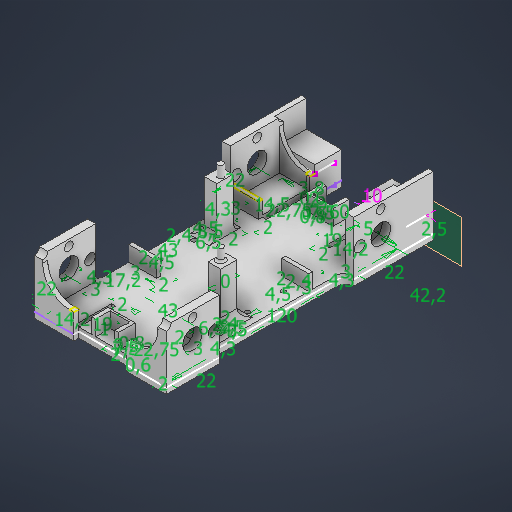
# Autodesk Inventor part: MainBody_thin
Saved by Autodesk Inventor 2026.1 (Build 301233000, 233)
## iProperties
Created: 2026-05-04
Part Number: MainBody_thin
Material: Generic
Document SubType Name: Modeling
Designer: 25adoh
Density: 1 g/cm^3
Appearance: Default
Author: 25adoh
Autodesk Inventor part; units mm, degrees
ref_plane "YZ Plane" through (0, 0, 0) normal (1, 0, 0) x (0, 1, 0)
ref_plane "XZ Plane" through (0, 0, 0) normal (0, 1, 0) x (-1, 0, 0)
ref_plane "XY Plane" through (0, 0, 0) normal (0, 0, 1) x (1, 0, 0)
sketch "Sketch1" plane through (0, 0, 0) normal (0, 1, 0) x (-1, 0, 0)
  line L0 (0, 0) -> (-60, 0)
  line L1 (-60, 0) -> (-60, -120)
  line L2 (-60, -120) -> (0, -120)
  line L3 (0, -120) -> (0, 0)
  line L4 (0, 0) -> (4.3, 0)
  line L5 (4.3, 0) -> (4.3, -22)
  line L6 (4.3, -22) -> (0, -22)
  line L7 (0, -22) -> (0, 0)
  line L8 (-60, 0) -> (-64.3, 0)
  line L9 (-64.3, 0) -> (-64.3, -22)
  line L10 (-64.3, -22) -> (-60, -22)
  line L11 (-60, -22) -> (-60, 0)
  line L12 (0, -120) -> (4.3, -120)
  line L13 (4.3, -120) -> (4.3, -98)
  line L14 (4.3, -98) -> (0, -98)
  line L15 (0, -98) -> (0, -120)
  line L16 (-60, -120) -> (-64.3, -120)
  line L17 (-64.3, -120) -> (-64.3, -98)
  line L18 (-64.3, -98) -> (-60, -98)
  line L19 (-60, -98) -> (-60, -120)
  line L20 (-45.8, -101.0095) -> (-43.8, -101.0095)
  line L21 (-43.8, -101.0095) -> (-43.8, -120)
  line L22 (-14.2, 0) -> (-14.2, -19)
  line L23 (-14.2, -19) -> (-16.2, -19)
  line L24 (-16.2, -19) -> (-16.2, 0)
  line L25 (-16.2, 0) -> (-14.2, 0)
  line L26 (-16.5, -120) -> (-14.5, -120)
  line L27 (-45.2, -120) -> (-43.8, -120)
  line L28 (-46, -77.8) -> (-60, -77.8)
  line L29 (-46, -77.8) -> (-46, -75.8)
  line L30 (-46, -75.8) -> (-60, -75.8)
  line L31 (0, 0) -> (-14.2, 0)
  line L32 (-14.5, -42.2) -> (0, -42.2)
  line L33 (-43.5, 0) -> (-43.5, -22.75)
  line L34 (-45.5, 0) -> (-45.5, -22.75)
  line L35 (-45.5, -22.75) -> (-43.5, -22.75)
  line L36 (-43.5, -22.75) -> (-43.5, -24.75)
  line L37 (-43.5, 0) -> (-45.5, 0)
  line L38 (-43.5, -24.75) -> (-60, -24.75)
  line L39 (-45.5, -22.75) -> (-60, -22.75)
  line L40 (-14.5, -120) -> (-14.5, -97.25)
  line L41 (-14.5, -97.25) -> (0, -97.25)
  line L42 (-16.5, -120) -> (-16.5, -97.25)
  line L43 (-16.5, -97.25) -> (-14.5, -97.25)
  line L44 (-16.5, -97.25) -> (-16.5, -95.25)
  line L45 (-16.5, -95.25) -> (0, -95.25)
  line L46 (-45.5, 0) -> (-45.5, 0.6)
  line L47 (-60, 0) -> (-60, 0.6)
  line L48 (-60, 0.6) -> (-45.5, 0.6)
  line L49 (-60, 0.6) -> (-60, 2.6)
  line L50 (-60, 2.6) -> (-43.5, 2.6)
  line L51 (-43.5, 2.6) -> (-43.5, 0)
  line L52 (-16.5, -120) -> (-16.5, -120.6)
  line L53 (-16.5, -120.6) -> (0, -120.6)
  line L54 (-16.5, -120.6) -> (-16.5, -122.6)
  line L55 (-16.5, -122.6) -> (0, -122.6)
  line L56 (0, -122.6) -> (0, -120.6)
  line L57 (0, -120.6) -> (0, -120)
  line L58 (-14.5, -120) -> (-14.5, -120.6)
  line L59 (-16.2, 0) -> (0, 0)
  line L60 (0, 0) -> (0, 2.6)
  line L61 (0, 2.6) -> (-16.2, 2.6)
  line L62 (-16.2, 2.6) -> (-16.2, 0)
  line L63 (-43.8, -120) -> (-59.8, -120)
  line L64 (-59.8, -120) -> (-59.8, -122.6)
  line L65 (-59.8, -122.6) -> (-43.8, -122.6)
  line L66 (-43.8, -122.6) -> (-43.8, -120)
  line L67 (-45.8, -101.0095) -> (-45.8, -120)
  line L68 (-14.5, -42.2) -> (-14.5, -44.2)
  line L69 (-14.5, -44.2) -> (0, -44.2)
  line L70 (-35, -120) -> (-35, 0)
  line L71 (-64.3, -22) -> (-60, -22)
  line L72 (-60, -22) -> (-60, -25)
  line L73 (-60, -25) -> (-64.3, -25)
  line L74 (-64.3, -25) -> (-64.3, -22)
  line L75 (-64.3, -98) -> (-60, -98)
  line L76 (-60, -98) -> (-60, -95)
  line L77 (-60, -95) -> (-64.3, -95)
  line L78 (-64.3, -95) -> (-64.3, -98)
  line L79 (4.3, -22) -> (0, -22)
  line L80 (0, -22) -> (0, -25)
  line L81 (0, -25) -> (4.3, -25)
  line L82 (4.3, -25) -> (4.3, -22)
  line L83 (4.3, -98) -> (0, -98)
  line L84 (0, -98) -> (0, -95)
  line L85 (0, -95) -> (4.3, -95)
  line L86 (4.3, -95) -> (4.3, -98)
  line L87 (-64.3, 0) -> (-60, 0)
  line L88 (-60, 0) -> (-60, 2.6)
  line L89 (-60, 2.6) -> (-64.3, 2.6)
  line L90 (-64.3, 2.6) -> (-64.3, 0)
  line L91 (0, 2.6) -> (4.3, 2.6)
  line L92 (4.3, 2.6) -> (4.3, 0)
  line L93 (4.3, 0) -> (0, 0)
  line L94 (0, 0) -> (0, 2.6)
  line L95 (0, -122.6) -> (4.3, -122.6)
  line L96 (4.3, -122.6) -> (4.3, -120)
  line L97 (4.3, -120) -> (0, -120)
  line L98 (0, -120) -> (0, -122.6)
  line L99 (-64.3, -120) -> (-59.8, -120)
  line L100 (-59.8, -120) -> (-59.8, -122.6)
  line L101 (-59.8, -122.6) -> (-64.3, -122.6)
  line L102 (-64.3, -122.6) -> (-64.3, -120)
  line L103 (-25, 0) -> (-35, 0)
  line L104 (-35, 0) -> (-35, -7.5)
  line L105 (-35, -7.5) -> (-25, -7.5)
  line L106 (-25, -7.5) -> (-25, 0)
  line L107 (-35, -7.5) -> (-35, -6.7)
  line L108 (-35, -5.7) -> (-35, -6.7)
  line L109 (-25, 0) -> (-23, 0)
  line L110 (-35, -7.5) -> (-37, -7.5)
  line L111 (-37, -7.5) -> (-37, 0)
  line L112 (-37, 0) -> (-35, 0)
  line L113 (-35, 0) -> (-35, -7.5)
  line L114 (-35, -6.7) -> (-35.3, -6.7)
  line L115 (-35, -6.5) -> (-35, -6.7)
  line L116 (-37, -7.5) -> (-23, -7.5)
  line L117 (-23, -8.5) -> (-37, -8.5)
  line L118 (-37, -8.5) -> (-37, -7.5)
  line L119 (-35, -6.7) -> (-35.5, -6.7)
  line L120 (-35.5, -6.7) -> (-35.5, -5.7)
  line L121 (-35.5, -5.7) -> (-35, -5.7)
  line L122 (-35, -5.7) -> (-35, -6.7)
  line L123 (-14.2, 0) -> (0, 0)
  line L124 (0, -25) -> (0, -42.2)
  line L125 (-23, -8.5) -> (-23, 0)
  line L126 (-25, -120) -> (-25, 0)
  circle A0 centre (-7, -69) radius 1.2
  circle A1 centre (-7, -51) radius 1.2
  circle A2 centre (-53.3, -50.7) radius 1.2
  circle A3 centre (-53.3, -69.3) radius 1.2
  line L127 (-51.5, -81.5) -> (-8.5, -81.5)
  line L128 (-8.5, -81.5) -> (-8.5, -38.5)
  line L129 (-8.5, -38.5) -> (-51.5, -38.5)
  line L130 (-51.5, -38.5) -> (-51.5, -81.5)
  line L131 (-51.5, -81.5) -> (-8.5, -38.5) construction
  line L132 (-8.5, -81.5) -> (-51.5, -38.5) construction
  circle A4 centre (-11.25, -41.25) radius 1.5
  circle A5 centre (-11.25, -41.25) radius 2.25
  line L133 (-9, -43.5) -> (-13.5, -43.5)
  line L134 (-13.5, -43.5) -> (-13.5, -39)
  line L135 (-13.5, -39) -> (-9, -39)
  line L136 (-9, -39) -> (-9, -43.5)
  circle A6 centre (-48.75, -41.25) radius 1.5
  circle A7 centre (-48.75, -41.25) radius 2.25
  line L137 (-51, -43.5) -> (-46.5, -43.5)
  line L138 (-46.5, -43.5) -> (-46.5, -39)
  line L139 (-46.5, -39) -> (-51, -39)
  line L140 (-51, -39) -> (-51, -43.5)
  circle A8 centre (-48.75, -78.75) radius 1.5
  circle A9 centre (-48.75, -78.75) radius 2.25
  line L141 (-46.5, -76.5) -> (-51, -76.5)
  line L142 (-51, -76.5) -> (-51, -81)
  line L143 (-51, -81) -> (-46.5, -81)
  line L144 (-46.5, -81) -> (-46.5, -76.5)
  circle A10 centre (-11.25, -78.75) radius 1.5
  circle A11 centre (-11.25, -78.75) radius 2.25
  line L145 (-13.5, -76.5) -> (-9, -76.5)
  line L146 (-9, -76.5) -> (-9, -81)
  line L147 (-9, -81) -> (-13.5, -81)
  line L148 (-13.5, -81) -> (-13.5, -76.5)
  line L149 (-14.5, -97.25) -> (-14.5, -95.25)
  line L150 (-45.5, -22.75) -> (-45.5, -24.75)
  line L151 (-46.5, -70.3) -> (-51, -70.3)
  line L152 (-51, -70.3) -> (-51, -65.8)
  line L153 (-51, -65.8) -> (-46.5, -65.8)
  line L154 (-46.5, -65.8) -> (-46.5, -70.3)
  line L155 (-13.5, -49.7) -> (-9, -49.7)
  line L156 (-9, -49.7) -> (-9, -54.2)
  line L157 (-9, -54.2) -> (-13.5, -54.2)
  line L158 (-13.5, -54.2) -> (-13.5, -49.7)
  line L159 (-25, -120) -> (-25, -112.5)
  line L160 (-25, -112.5) -> (-35, -112.5)
  line L161 (-35, -112.5) -> (-35, -120)
  line L162 (-25, -112.5) -> (-25, -113.3)
  line L163 (-25, -114.3) -> (-25, -113.3)
  line L164 (-35, -120) -> (-37, -120)
  line L165 (-25, -112.5) -> (-23, -112.5)
  line L166 (-23, -112.5) -> (-23, -120)
  line L167 (-23, -120) -> (-25, -120)
  line L168 (-25, -120) -> (-25, -112.5)
  line L169 (-25, -113.3) -> (-24.7, -113.3)
  line L170 (-25, -113.5) -> (-25, -113.3)
  line L171 (-23, -112.5) -> (-37, -112.5)
  line L172 (-37, -111.5) -> (-23, -111.5)
  line L173 (-23, -111.5) -> (-23, -112.5)
  line L174 (-25, -113.3) -> (-24.5, -113.3)
  line L175 (-24.5, -113.3) -> (-24.5, -114.3)
  line L176 (-24.5, -114.3) -> (-25, -114.3)
  line L177 (-25, -114.3) -> (-25, -113.3)
  line L178 (-37, -111.5) -> (-37, -120)
  line L179 (-30, -60) -> (-30, -60)
  line L180 (-30, -60) -> (-30, -60)
  line L181 (-30, -60) -> (-30, -60)
  line L182 (-53.3, -120) -> (-53.1894, -77.8)
  line L183 (-64.3, -122.6) -> (-42.6503, -122.6)
  line L184 (-64.3, -122.6) -> (-59.3, -122.6)
  line L185 (-47.6503, -122.6) -> (-42.6503, -122.6)
  line L186 (4.3, -122.6) -> (-16.5, -122.6)
  line L187 (4.3, -132.6) -> (4.3, -122.6)
  line L188 (-16.5, -122.6) -> (-11.5, -122.6)
  line L189 (4.3, -122.6) -> (-0.7, -122.6)
  line L190 (4.3, -132.6) -> (4.3, -122.6)
  line L191 (-46.5, -43.5) -> (-46.5, -45.5)
  line L192 (-46.5, -45.5) -> (-53, -45.5)
  line L193 (-53, -45.5) -> (-53, -37)
  line L194 (-53, -37) -> (-46.5, -37)
  line L195 (-46.5, -37) -> (-46.5, -45.5)
  line L196 (-13.5, -81) -> (-13.5, -83)
  line L197 (-13.5, -83) -> (-7, -83)
  line L198 (-7, -83) -> (-7, -74.5)
  line L199 (-7, -74.5) -> (-13.5, -74.5)
  line L200 (-13.5, -74.5) -> (-13.5, -83)
  line L201 (-64.3, -120) -> (4.3, -120)
  line L202 (4.3, -120) -> (4.3, -136.4)
  line L203 (-0.7, -122.6) -> (-11.5, -122.6)
  line L204 (-11.5, -122.6) -> (-11.5, -126.4)
  line L205 (-11.5, -126.4) -> (-0.7, -126.4)
  line L206 (-0.7, -126.4) -> (-0.7, -122.6)
  line L207 (-16.5, -136.4) -> (-11.5, -136.4)
  line L208 (-11.5, -136.4) -> (-11.5, -122.6)
  line L209 (-11.5, -122.6) -> (-16.5, -122.6)
  line L210 (-16.5, -122.6) -> (-16.5, -136.4)
  line L211 (4.3, -136.4) -> (-0.7, -136.4)
  line L212 (-0.7, -136.4) -> (-0.7, -122.6)
  line L213 (-0.7, -122.6) -> (4.3, -122.6)
  line L214 (4.3, -122.6) -> (4.3, -136.4)
  line L215 (-0.7, -136.4) -> (-11.5, -136.4)
  line L216 (-64.3, -122.6) -> (-59.8, -122.6)
  line L217 (-59.8, -122.6) -> (-59.8, -136.4)
  line L218 (-59.8, -136.4) -> (-64.3, -136.4)
  line L219 (-64.3, -136.4) -> (-64.3, -122.6)
  line L220 (-42.6503, -122.6) -> (-47.6503, -122.6)
  line L221 (-47.6503, -122.6) -> (-47.6503, -136.4)
  line L222 (-47.6503, -136.4) -> (-42.6503, -136.4)
  line L223 (-42.6503, -136.4) -> (-42.6503, -122.6)
  line L224 (-47.6503, -136.4) -> (-59.8, -136.4)
  line L225 (-47.6503, -126.4) -> (-59.8, -126.4)
  line L226 (-42.6503, -122.6) -> (-42.6503, -120)
  line L227 (-64.3, -120) -> (-61.8, -120)
  line L228 (-61.8, -120) -> (-61.8, -136.4)
  line L229 (-61.8, -136.4) -> (-64.3, -136.4)
  line L230 (-64.3, -136.4) -> (-64.3, -120)
  line L231 (4.3, -122.6) -> (1.8, -122.6)
  line L232 (1.8, -122.6) -> (1.8, -136.4)
  line L233 (1.8, -136.4) -> (4.3, -136.4)
  line L234 (4.3, -136.4) -> (4.3, -122.6)
  line L235 (1.8, -122.6) -> (4.3, -122.6)
  line L236 (4.3, -122.6) -> (4.3, -120)
  line L237 (4.3, -120) -> (1.8, -120)
  line L238 (1.8, -120) -> (1.8, -122.6)
  point P0 (-60, -98)
  point P1 (0, -98)
  point P2 (0, -29.2)
  point P3 (-35, -130)
  point P4 (-45.8, -120)
  point P5 (-60, -120)
  point P6 (-30, -70)
  point P7 (-30, -60)
  point P8 (-30, -60)
  point P9 (-12.75, -42.75)
  point P10 (-35, -8.5)
  point P11 (-25, -120)
  point P12 (-37, -120)
  point P13 (-35, -112.5)
  point P14 (-25, -112.5)
  point P15 (-25, -113.3)
  point P16 (-25, -114.3)
  point P17 (-23, -120)
  point P18 (-25, -120)
  point P19 (-25, -111.5)
  point P20 (-25, -112.5)
  point P21 (-25, -120)
  point P22 (-35, -111.5)
  point P23 (-16.5, -132.6)
  point P24 (-51, -41.25)
  point P25 (-43.8, -122.6)
  point P26 (-0.7, -126.4)
  point P27 (-0.7, -122.6)
  dimension "d0" = 60
  dimension "d1" = 120
  dimension "d2" = 4.3
  dimension "d3" = 22
  dimension "d4" = 4.3
  dimension "d5" = 22
  dimension "d6" = 4.3
  dimension "d7" = 22
  dimension "d8" = 4.3
  dimension "d9" = 22
  dimension "d66" = 19
  dimension "d67" = 2
  dimension "d74" = 19
  dimension "d75" = 2
  dimension "d100" = 2
  dimension "d107" = 22.75
  dimension "d108" = 2
  dimension "d109" = 22.75
  dimension "d110" = 2
  dimension "d111" = 0.6
  dimension "d112" = 2
  dimension "d113" = 0.6
  dimension "d114" = 2
  dimension "d148" = 2
  dimension "d165" = 3
  dimension "d166" = 3
  dimension "d167" = 3
  dimension "d168" = 3
  dimension "d175" = 7.5
  dimension "d176" = 0.8
  dimension "d180" = 2
  dimension "d182" = 1
  dimension "d183" = 0.5
  dimension "d186" = 14.2
  dimension "d190" = 17.2
  dimension "d196" = 2.4
  dimension "d197" = 2.4
  dimension "d198" = 2.4
  dimension "d199" = 43
  dimension "d200" = 43
  dimension "d201" = 3
  dimension "d202" = 3
  dimension "d203" = 4.5
  dimension "d204" = 3
  dimension "d205" = 4.5
  dimension "d206" = 4.5
  dimension "d207" = 4.5
  dimension "d209" = 2.4
  dimension "d215" = 7.5
  dimension "d216" = 0.8
  dimension "d217" = 2
  dimension "d218" = 1
  dimension "d219" = 0.5
  dimension "d224" = 0
  dimension "d225" = 42.2
  dimension "d228" = 5
  dimension "d238" = 2
  dimension "d239" = 6.5
  dimension "d240" = 8.5
  dimension "d241" = 2
  dimension "d242" = 6.5
  dimension "d243" = 8.5
  dimension "d247" = 14.2
  dimension "d248" = 14.5
  constraints: 474 end point, 79 parallel, 57 perpendicular, 53 horizontal, 27 point on line, 20 vertical, 12 centre point, 4 coincident, 4 midpoint, 3 collinear, 20 other
  measures "d0" distance of L2.end L1.end
  measures "d1" distance of L1.end L1.start
  measures "d2" distance of L5.end L6.end
  measures "d3" distance of L4.end L5.end
  measures "d4" distance of L10.end L9.end
  measures "d5" distance of L9.end L8.end
  measures "d6" distance of L14.end L13.end
  measures "d7" distance of L13.end L12.end
  measures "d8" distance of L17.end L18.end
  measures "d9" distance of L16.end L17.end
  measures "d66" distance of L27.start L20.start
  measures "d67" distance of L20.start L20.end
  measures "d74" distance of L22.start L22.end
  measures "d75" distance of L22.end L23.end
  measures "d100" distance of L28.start L29.end
  measures "d107" distance of L33.start L33.end
  measures "d108" distance of L33.end L36.end
  measures "d109" distance of L26.end L40.end
  measures "d110" distance of L42.end L44.end
  measures "d111" distance of L34.start L46.end
  measures "d112" distance of L47.end L49.end
  measures "d113" distance of L26.start L52.end
  measures "d114" distance of L52.end L54.end
  measures "d148" distance of L32.start L68.end
  measures "d165" distance of L71.end L72.end
  measures "d166" distance of L76.end L75.end
  measures "d167" distance of L80.end L79.end
  measures "d168" distance of L83.end L84.end
  measures "d175" distance of L104.end L103.end
  measures "d176" distance of L104.end L107.end
  measures "d180" distance of L111.end L112.end
  measures "d182" distance of L116.end L117.start
  measures "d183" distance of L120.end L121.end
  measures "d186" distance of L4.start L22.start
  measures "d190" distance of L80.end L32.end
  measures "d196" diameter of A0
  measures "d197" diameter of A2
  measures "d198" diameter of A3
  measures "d199" distance of L129.end L128.end
  measures "d200" distance of L128.end L127.end
  measures "d201" diameter of A4
  measures "d202" diameter of A6
  measures "d203" diameter of A7
  measures "d204" diameter of A8
  measures "d205" diameter of A11
  measures "d206" distance of L151.end L152.end
  measures "d207" distance of L155.end L156.end
  measures "d209" diameter of A1
  measures "d215" distance of L160.start L159.start
  measures "d216" distance of L160.start L177.end
  measures "d217" distance of L167.start L168.start
  measures "d218" distance of L171.end L178.start
  measures "d219" distance of L175.end L177.start
  measures "d224" distance of L180.end L181.end
  measures "d225" vertical distance of L182.start L182.end
  measures "d228" distance of L185.start L185.end
  measures "d238" distance of L137.end L191.end
  measures "d239" distance of L193.end L194.end
  measures "d240" distance of L192.end L193.end
  measures "d241" distance of L148.start L196.end
  measures "d242" distance of L199.end L198.end
  measures "d243" distance of L198.end L197.end
  measures "d247" distance between parallel lines of L67 L1
  measures "d248" distance between parallel lines of L40 L15
extrude "Extrusion1" add sketch "Sketch1" along normal blind 2 and the other way blind 3 contours L3 L32 L128 L129 L126 L117 L125 L0 L24 L23 L22 | L22 L23 L24 L0 | L125 L116 L106 L0 | L3 L69 L128 L32 | L106 L105 L70 L0 | L125 L117 L126 L116 | L3 L45 L44 L42 L2 L166 L173 L172 L126 L127 L196 L197 L198 L199 L128 L69 | L128 L69 L68 L32 L134 L133 L136 | L32 L136 L135 L134 L68 L69 L128 L199 L200 L148 L196 L127 L126 L129 | L70 L121 L120 L119 L114 L110 L111 L0 | L126 L117 L70 L105 | L136 L133 A5 L32 | L32 A5 L136 | L111 L118 L117 L70 L129 L195 L194 L193 L192 L130 L30 L1 L38 L36 L33 L0 | L70 L114 L119 L120 L121 | L70 L117 L118 L110 | L126 L129 L70 L117 | L3 L41 L149 L45 | L199 L198 L197 L196 L127 L128 | L128 L127 L196 L147 L146 L145 L200 L199 | A5 L32 A4 | L32 A4 A5 | A5 L135 L136 | L126 L127 L70 L129 | L33 L35 L34 L0 | L0 L46 L48 L49 L50 L51 | L3 L2 L40 L41 | L149 L43 L44 L45 | A4 L32 | L32 A4 | L133 L134 L32 A5 | A5 L134 L135 | L126 L172 L70 L127 | L70 L127 L130 L28 L142 L143 L144 L29 L30 L192 L191 L138 L195 L129 | L34 L39 L1 L0 | L0 L47 L48 L46 | L36 L38 L150 L35 | L40 L2 L42 L43 | L134 A5 L32 | L145 A11 L148 | L172 L173 L165 L126 | L126 L160 L70 L172 | L70 L172 L178 L2 L21 L20 L67 L182 L28 L130 L127 | L195 L139 L140 L137 L191 L192 L130 L129 | L129 L130 L192 L193 L194 L195 | L150 L38 L1 L39 | L57 L53 L58 L2 | L58 L53 L52 L2 | L187 L202 L211 L232 L95 | L148 A11 L147 | L145 L146 A11 | A11 | L165 L166 L2 L126 L176 L175 L174 L169 | L126 L2 L70 L160 | L70 L171 L178 L172 | L138 A7 L139 | L56 L55 L54 L53 | L232 L211 L212 L206 L55 L95 | A11 L146 L147 | L169 L174 L175 L176 L126 | L70 L2 L178 L171 | L130 L30 L29 L28 L144 L141 L142 | L28 L1 L30 L130 | A7 | L138 L137 A7 | A7 L140 L139 | L142 L141 A9 L28 | L28 A9 L142 | L182 L2 L1 L28 | L137 L140 A7 | L55 L204 L208 L207 L210 | A9 L28 A8 | L28 A8 A9 | A9 L143 L142 | A8 L28 | L28 A8 | L141 L144 L28 A9 | A9 L144 L143 | L67 L20 L21 L2 | L223 L222 L221 L65 L183 | L28 L144 A9 | L217 L218 L228 L101 | L228 L218 L219 L101 | A0 | A1 | A2 | A3 | A6 | A10 | L151 L152 L153 L154 | L155 L156 L157 L158
extrude "Extrusion2" add sketch "Sketch1" along normal blind 28 and the other way blind 3 contours L4 L5 L6 L3 | L6 L82 L81 L3 | L85 L86 L14 L3 | L13 L12 L3 L14 | L96 L95 L238 L12 | L1 L10 L9 L8 | L187 L202 L211 L232 L95 | L1 L73 L74 L10 | L1 L18 L78 L77 | L1 L16 L17 L18 | L228 L101 L102 L16 | L228 L218 L219 L101
sketch "Sketch2" plane through (64.3, -3, 0) normal (1, 0, 0) x (0, 0, -1)
  line L0 (0, 31) -> (25, 31) projected
  line L1 (22, 0) -> (22, 28) projected
  line L2 (0, 31) -> (0, 8)
  line L3 (0, 8) -> (22, 8)
  line L4 (0, 31) -> (22, 8)
  line L5 (22, 0) -> (22, 28) projected
  line L6 (0, 8) -> (22, 28)
  circle A0 centre (11, 18) radius 5.1
  line L7 (98, 28) -> (120, 28)
  line L8 (98, 0) -> (98, 28)
  line L9 (120, 0) -> (120, 28)
  line L10 (98, 28) -> (98, 5)
  line L11 (98, 5) -> (120, 5)
  line L12 (98, 28) -> (120, 5)
  line L13 (120, 0) -> (120, 28)
  line L14 (98, 5) -> (120, 28)
  circle A1 centre (109, 16.5) radius 5.1
  line L15 (120, 31) -> (120, 0) projected
  line L16 (0, 31) -> (0, 8)
  line L17 (12.5, 31) -> (11.25, 31) construction
  circle A2 centre (11, 27.75) radius 2.25
  circle A3 centre (109, 27.75) radius 2.25
  circle A4 centre (22, 16.5) radius 2.75
  circle A5 centre (98, 16.5) radius 2.75
  point P0 (118, 16.5)
  dimension "d14" = 23
  dimension "d15" = 10.2
  dimension "d16" = 23
  dimension "d17" = 10.2
  dimension "d60" = 4.5
  dimension "d61" = 4.5
  dimension "d115" = 5.5
  dimension "d214" = 5.5
  constraints: 28 end point, 6 centre point, 4 point on line, 3 midpoint, 3 perpendicular, 1 coincident, 1 horizontal, 2 other
  measures "d14" distance of L2.start L2.end
  measures "d15" diameter of A0
  measures "d16" distance of L7.start L10.end
  measures "d17" diameter of A1
  measures "d60" diameter of A2
  measures "d61" diameter of A3
  measures "d115" diameter of A4
  measures "d214" diameter of A5
extrude "Extrusion3" cut sketch "Sketch2" against normal up to surface (68.6 mm away) contours A4 L1 | L1 A4 | A0 L6 L4 | L4 L6 A0 | A0 L4 L6 | L4 A0 L6 | A3 L7 | L7 A3 | A5 L8 | L8 A5 | A1 L14 L12 | L12 L14 A1 | L14 A1 L12 | L12 A1 L14 | A2
ref_plane "Work Plane1" through (64.5, 0, -140) normal (0, 0, -1) x (-1, 0, 0)
sketch "Sketch5" plane through (64.5, 0, -140) normal (0, 0, -1) x (-1, 0, 0)
  line L0 (42, 5) -> (42, 20) projected
  line L1 (4.5, 2) -> (4.5, 28) projected
  line L2 (2.7, 28) -> (4.5, 28) projected
  line L3 (34.5, 20) -> (34.5, 5)
  line L4 (27, 5) -> (42, 5) projected
  line L5 (34.5, 5) -> (34.5, 13)
  line L6 (30.5, 13) -> (38.5, 13)
  line L7 (38.5, 13) -> (38.5, 5)
  line L8 (30.5, 13) -> (30.5, 5)
  line L9 (48, -3) -> (48, 2) projected
  line L10 (4.5, 2) -> (48, 2) projected
  line L11 (48, -3) -> (2.7, -3) projected
  line L12 (2.7, 28) -> (2.7, -3) projected
  point P0 (64.5, 0)
  point P1 (42, 5)
  dimension "d40" = 8
  dimension "d41" = 8
  constraints: 10 end point, 3 point on line, 2 midpoint, 2 perpendicular, 1 horizontal
  measures "d40" distance of L3.end L5.end
  measures "d41" distance of L6.start L6.end
extrude "Extrusion6" cut sketch "Sketch5" against normal blind 6 contours L6 L7 L4 L3 | L3 L4 L8 L6
extrude "Extrusion7" add sketch "Sketch1" along normal blind 10 and the other way blind 3 contours L60 L91 L92 L4 | L0 L62 L61 L60 | L3 L69 L128 L32 | L128 L69 L68 L32 L134 L133 L136 | L136 L133 A5 L32 | L3 L41 L149 L45 | A5 L32 A4 | L0 L46 L48 L49 L50 L51 | A4 L32 | L133 L134 L32 A5 | L96 L95 L238 L12 | L8 L90 L89 L49 L47 | L150 L38 L1 L39 | L12 L238 L95 L56 L57 | L58 L53 L52 L2 | L56 L55 L54 L53 | L130 L30 L29 L28 L144 L141 L142 | L28 L1 L30 L130 | L142 L141 A9 L28 | A9 L28 A8 | L2 L66 L65 L64 | A8 L28 | L141 L144 L28 A9 picked at (-12.908, -42.3449) picked at (-10.942, -42.2772) picked at (-50.408, -77.6551) picked at (-49.043, -77.5876)
extrude "Extrusion8" add sketch "Sketch1" along normal blind 28 contours L199 L198 L197 L196 L127 L128 | L128 L127 L196 L147 L146 L145 L200 L199 | L145 A11 L148 | L195 L139 L140 L137 L191 L192 L130 L129 | L129 L130 L192 L193 L194 L195 | L148 A11 L147 | L145 L146 A11 | A11 | L138 A7 L139 | A11 L146 L147 | A7 | L138 L137 A7 | A7 L140 L139 | L137 L140 A7 | A6 | A10
extrude "Extrusion9" add sketch "Sketch1" along normal blind 34 contours A6 | A10
fillet "Fillet3" radius 4.5 4 edges at (0, -0.5, -25) (0, -0.5, -95) (60, -0.5, -95) (60, -0.5, -25)
extrude "Extrusion12" add sketch "Sketch1" along normal blind 3 contours L3 L2 L40 L41 | L34 L39 L1 L0 | L0 L47 L48 L46 | L57 L53 L58 L2
extrude "Extrusion14" cut sketch "Sketch1" along normal blind 5 and the other way blind 5 contours A0 | A1 | A2 | A3
fillet "Fillet4" radius 1.5 4 edges at (54.5, -3, -50.7) (54.5, -3, -69.3) (8.2, -3, -51) (8.2, -3, -69)
fillet "Fillet5" radius 4 6 edges at (53, 2, -41.25) (49.75, 2, -37) (49.75, 2, -45.5) (10.25, 2, -74.5) (10.25, 2, -83) (7, 2, -78.75)
extrude "Extrusion15" add sketch "Sketch1" along normal blind 25.4 and the other way blind 3 contours L60 L91 L92 L4 | L96 L95 L238 L12 | L8 L90 L89 L49 L47 | L12 L238 L95 L56 L57 | L64 L101 L228 L16 L2 | L228 L101 L102 L16
fillet "Fillet6" radius 2.6 4 edges at (-2.15, 25.4, 0) (62.15, 25.4, 0) (-0.9, 25.4, -120) (60.9, 25.4, -120)
fillet "Fillet7" radius 14 4 edges at (60, 10, 1.6) (0, 10, 1.3) (0, 10, -121.6) (59.8, 10, -121.3)
extrude "Extrusion16" add sketch "Sketch1" along normal blind 10 contours L125 L116 L106 L0 | L125 L117 L126 L116 | L70 L121 L120 L119 L114 L110 L111 L0 | L126 L117 L70 L105 | L70 L117 L118 L110 | L172 L173 L165 L126 | L126 L160 L70 L172 | L165 L166 L2 L126 L176 L175 L174 L169 | L70 L171 L178 L172 | L70 L2 L178 L171
extrude "Extrusion17" add sketch "Sketch1" along normal blind 4 and the other way blind 3 contours L206 L205 L204 L55 | L215 L208 L205 L212 | L65 L221 L225 L217 | L225 L221 L224 L217
sketch "Sketch7" plane through (0, 10, 0) normal (0, 1, 0) x (1, 0, 0)
  line L0 (42.6503, 122.6) -> (42.6503, 132.6) projected
  line L1 (64.3, 132.6) -> (42.6503, 132.6)
  line L2 (42.6503, 132.6) -> (42.6503, 122.6)
  line L3 (42.6503, 122.6) -> (64.3, 122.6)
  line L4 (64.3, 122.6) -> (64.3, 132.6)
  line L5 (16.5, 122.6) -> (14, 122.6) projected
  line L6 (16.5, 122.6) -> (16.5, 120) projected
  line L7 (-4.3, 132.6) -> (16.5, 132.6)
  line L8 (16.5, 132.6) -> (16.5, 122.6)
  line L9 (16.5, 122.6) -> (-4.3, 122.6)
  line L10 (-4.3, 122.6) -> (-4.3, 132.6)
  line L11 (0, 95.25) -> (0, 97.25) projected
  line L12 (14, 120.6) -> (14.5, 120.6) projected
  line L13 (14.5, 120.6) -> (14.5, 120) projected
  line L14 (14.5, 120) -> (16.5, 120) projected
  line L15 (16.5, 120) -> (16.5, 122.6) projected
  line L16 (14.5, 97.25) -> (0, 97.25) projected
  line L17 (0, 95.25) -> (14.5, 95.25) projected
  line L18 (14.5, 95.25) -> (14.5, 97.25) projected
  line L19 (14, -2.6) -> (16.2, -2.6) projected
  line L20 (16.2, -2.6) -> (16.2, 0) projected
  line L21 (16.2, 0) -> (14, 0) projected
  line L22 (14, -2.6) -> (14, 0) projected
  line L23 (14, 120.6) -> (14, 122.6) projected
  point P0 (0, 0)
  point P1 (42.6503, 132.6)
  point P2 (42.8503, 120)
  point P3 (16.5, 132.6)
  point P4 (16.5, 132.6)
  dimension "d234" = 10
  constraints: 17 end point, 4 parallel, 2 horizontal, 2 perpendicular, 2 other
  measures "d234" distance of L2.end L1.end
fillet "Fillet8" radius 1 1 edges at (50.25, 28, -41.25)
extrude "Extrusion19" cut sketch "Sketch1" along normal blind 2 and the other way blind 1 contours L22 L23 L24 L0 | L33 L35 L34 L0 | L40 L2 L42 L43 | L67 L20 L21 L2
extrude "Extrusion20" add sketch "Sketch1" along normal blind 10 and the other way blind 3 contours L187 L202 L211 L232 L95 | L232 L211 L212 L206 L55 L95 | L55 L204 L208 L207 L210 | L223 L222 L221 L65 L183 | L217 L218 L228 L101 | L228 L218 L219 L101
sketch "Sketch8" plane through (0, 10, 0) normal (0, 1, 0) x (1, 0, 0)
  line L0 (61.8, 136.4) -> (59.8, 136.4) projected
  line L1 (59.8, 136.4) -> (59.8, 122.6) projected
  line L2 (61.8, 122.6) -> (59.8, 122.6) projected
  line L3 (11.5, 136.4) -> (11.5, 122.6) projected
  line L4 (14, 120.6) -> (14, 122.6) projected
  line L5 (14, 120.6) -> (14.5, 120.6) projected
  line L6 (14.5, 120.6) -> (14.5, 120) projected
  line L7 (14.5, 120) -> (16.5, 120) projected
  line L8 (16.5, 120) -> (16.5, 136.4) projected
  line L9 (16.5, 136.4) -> (11.5, 136.4) projected
  line L10 (11.5, 136.4) -> (11.5, 122.6) projected
  line L11 (14, 122.6) -> (11.5, 122.6) projected
  line L12 (0.7, 122.6) -> (-1.8, 122.6) projected
  line L13 (0.7, 122.6) -> (0.7, 136.4) projected
  line L14 (0.7, 136.4) -> (-1.8, 136.4) projected
  line L15 (-4.3, 136.4) -> (16.5, 136.4)
  line L16 (16.5, 136.4) -> (16.5, 122.6)
  line L17 (16.5, 122.6) -> (-4.3, 122.6)
  line L18 (-4.3, 122.6) -> (-4.3, 136.4)
  line L19 (45.8, 122.6) -> (45.8, 120) projected
  line L20 (47.6503, 122.6) -> (45.8, 122.6) projected
  line L21 (47.6503, 122.6) -> (47.6503, 136.4) projected
  line L22 (47.6503, 136.4) -> (42.6503, 136.4) projected
  line L23 (42.6503, 136.4) -> (42.6503, 122.6) projected
  line L24 (42.6503, 122.6) -> (43.8, 122.6) projected
  line L25 (43.8, 122.6) -> (43.8, 120) projected
  line L26 (43.8, 120) -> (45.8, 120) projected
  line L27 (42.6503, 136.4) -> (42.6503, 122.6) projected
  line L28 (42.6503, 136.4) -> (64.3, 136.4)
  line L29 (64.3, 136.4) -> (64.3, 122.6)
  line L30 (64.3, 122.6) -> (42.6503, 122.6)
  line L31 (42.6503, 122.6) -> (42.6503, 136.4)
  line L32 (-1.8, 122.6) -> (-1.8, 136.4) projected
  line L33 (61.8, 136.4) -> (61.8, 122.6) projected
  point P0 (0, 0)
  constraints: 16 end point, 4 parallel, 2 horizontal, 2 perpendicular, 1 point on line
extrude "Extrusion21" add sketch "Sketch8" along normal blind 4 contours L33 L2 L1 L0 | L28 L29 L30 L33 | L1 L30 L21 L28 | L21 L20 L30 L24 L23 L22 | L9 L8 L17 L11 L3 | L3 L17 L13 L15 | L13 L12 L32 L14 | L32 L17 L18 L15
body "Solid1"
